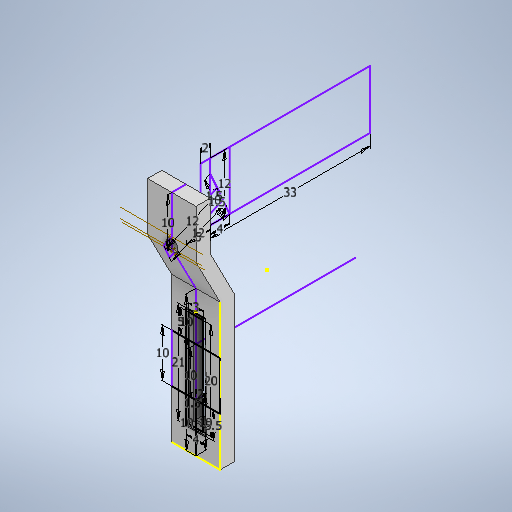
# Autodesk Inventor part: micro_wheel_mount
Saved by Autodesk Inventor 2025 (Build 290162000, 162)
## iProperties
Created: 2025-12-07
Part Number: micro_wheel_mount
Material: Типовые
Document SubType Name: Modeling
Designer: Admin
Density: 1 g/cm^3
Appearance: По умолчанию
Author: Admin
Autodesk Inventor part; units mm, degrees
ref_plane "YZ Plane" through (0, 0, 0) normal (1, 0, 0) x (0, 1, 0)
ref_plane "XZ Plane" through (0, 0, 0) normal (0, 1, 0) x (-1, 0, 0)
ref_plane "XY Plane" through (0, 0, 0) normal (0, 0, 1) x (1, 0, 0)
sketch "Эскиз1" plane through (0, 0, 0) normal (1, 0, 0) x (0, 1, 0)
  line L0 (13.9581, 11.7453) -> (25.9581, 11.7453)
  line L1 (25.9581, 11.7453) -> (25.9581, 13.7453)
  line L2 (25.9581, 13.7453) -> (13.9581, 13.7453)
  line L3 (13.9581, 13.7453) -> (13.9581, 11.7453)
  line L4 (13.9581, 11.7453) -> (13.9581, -21.2547)
  line L5 (13.9581, -21.2547) -> (25.9581, -21.2547)
  line L6 (25.9581, -21.2547) -> (25.9581, 11.7453)
  line L7 (13.9581, 11.7453) -> (13.9581, 7.7453)
  line L8 (13.9581, 7.7453) -> (25.9581, 7.7453)
  line L9 (-6.8518, -18.2547) -> (-6.8518, 11.7453)
  line L10 (-6.8518, 11.7453) -> (-15.825, 11.7453)
  line L11 (-15.825, 11.7453) -> (-15.825, 14.7104)
  line L12 (-15.825, 14.7104) -> (-5.825, 14.7104)
  line L13 (-5.825, 14.7104) -> (-5.825, 11.7453)
  line L14 (-15.825, 14.7104) -> (-25.825, 14.7104)
  line L15 (-25.825, 14.7104) -> (-25.825, 11.7453)
  line L16 (-15.825, 11.7453) -> (-25.825, 11.7453)
  line L17 (-5.825, 14.7104) -> (4.175, 14.7104)
  line L18 (4.175, 14.7104) -> (4.175, 11.7453)
  line L19 (13.9581, 7.7453) -> (23.1232, 11.7453)
  line L20 (23.1232, 11.7453) -> (18.5407, 9.7453)
  line L21 (18.5407, 9.7453) -> (19.9154, 10.3453)
  line L22 (18.5407, 9.7453) -> (17.1659, 9.1453)
  line L23 (19.9154, 10.3453) -> (15.1154, 21.3434)
  line L24 (17.1659, 9.1453) -> (12.3659, 20.1434)
  line L25 (12.3659, 20.1434) -> (15.1154, 21.3434)
  line L26 (13.9581, 11.7453) -> (13.8495, 16.7441)
  line L27 (13.8495, 16.7441) -> (4.175, 11.7453)
  line L28 (4.175, 14.7104) -> (13.7858, 19.6763)
  line L29 (13.7858, 19.6763) -> (23.7858, 19.6763)
  line L30 (23.7858, 19.6763) -> (23.7858, 16.7441)
  line L31 (23.7858, 16.7441) -> (13.8495, 16.7441)
  line L32 (4.175, 11.7453) -> (-5.825, 11.7453)
  line L33 (-5.825, 11.7453) -> (-6.8518, 11.7453)
  point P0 (0, 0)
  dimension "d0" = 12
  dimension "d1" = 2
  dimension "d2" = 33
  dimension "d3" = 4
  dimension "d4" = 10
  dimension "d5" = 10
  dimension "d6" = 10
  dimension "d7" = 10
  dimension "d8" = 1.5
  dimension "d9" = 1.5
  dimension "d10" = 12
  dimension "d11" = 12
  dimension "d12" = 5
  dimension "d13" = 10
  constraints: 68 end point, 11 perpendicular, 11 point on line, 3 horizontal, 2 vertical, 1 midpoint, 1 parallel
  measures "d0" distance of L7.start L6.end
  measures "d1" distance of L6.end L1.end
  measures "d2" distance of L7.start L4.end
  measures "d3" distance of L7.start L7.end
  measures "d4" distance of L11.end L13.start
  measures "d5" distance of L11.end L14.end
  measures "d6" distance of L13.start L18.start
  measures "d7" distance of L7.end L19.end
  measures "d8" distance of L22.start L21.end
  measures "d9" distance of L22.start L22.end
  measures "d10" distance of L21.end L23.end
  measures "d11" distance of L22.end L24.end
  measures "d12" distance of L7.start L31.end
  measures "d13" distance of L29.start L29.end
extrude "Выдавливание1" add sketch "Эскиз1" along normal blind 5 and the other way blind 5 contours L31 L24 L28 L29 L23 | L23 L29 L30 L31 | L27 L18 L28 L24 | L32 L13 L17 L18 | L33 L10 L11 L12 L13 | L11 L16 L15 L14
sketch "Эскиз2" plane through (-5, 4.175, 14.7104) normal (0, -0.459, 0.8884) x (1, 0, 0)
  line L0 (5, 9.6975) -> (5, 12.6658)
  line L1 (5, 12.6658) -> (5, 11.1658)
  circle A0 centre (5, 11.1658) radius 1.25
  point P0 (5, -10.4618)
  dimension "d18" = 1.5
  dimension "d19" = 2.5
  constraints: 4 end point, 1 centre point, 1 coincident, 1 point on line, 1 vertical
  measures "d18" distance of L0.end L1.end
  measures "d19" diameter of A0
sketch "Эскиз3" plane through (-5, -25.825, 14.7104) normal (0, 0, 1) x (1, 0, 0)
  line L0 (0, 0) -> (10, 0) projected
  line L1 (5, 0) -> (5, 10)
  line L2 (5, 10) -> (0, 10)
  line L3 (0, 10) -> (0, 20)
  line L4 (0, 20) -> (10, 20)
  line L5 (10, 20) -> (10, 10)
  line L6 (10, 30) -> (10, 0) projected
  line L7 (5, 10) -> (10, 10)
  line L8 (5, 10) -> (3.5, 10)
  line L9 (3.5, 10) -> (3.5, 20)
  line L10 (3.5, 20) -> (3.5, 25)
  line L11 (3.5, 25) -> (6.5, 25)
  line L12 (6.5, 25) -> (6.5, 5)
  line L13 (6.5, 5) -> (3.5, 5)
  line L14 (3.5, 5) -> (3.5, 10)
  line L15 (5, 10) -> (7, 10)
  line L16 (7, 10) -> (7, 4.5)
  line L17 (7, 4.5) -> (3, 4.5)
  line L18 (3, 4.5) -> (3, 25.5)
  line L19 (3, 25.5) -> (7, 25.5)
  line L20 (7, 25.5) -> (7, 10)
  line L21 (7, 10) -> (7, 4.5)
  line L22 (7, 4.5) -> (5, 4.5)
  line L23 (5, 4.5) -> (5, 10)
  line L24 (6.5, 10) -> (5, 10)
  line L25 (5, 10) -> (5, 5)
  line L26 (5, 5) -> (6.5, 5)
  line L27 (6.5, 5) -> (6.5, 10)
  point P0 (5, 25.825)
  point P1 (5, 5)
  point P2 (5, 5)
  dimension "d22" = 10
  dimension "d23" = 10
  dimension "d24" = 1.5
  dimension "d25" = 5
  dimension "d26" = 3
  dimension "d27" = 20
  dimension "d28" = 2
  dimension "d29" = 5.5
  dimension "d30" = 4
  dimension "d31" = 21
  constraints: 52 end point, 14 perpendicular, 10 point on line, 3 midpoint, 3 parallel, 2 collinear, 1 horizontal, 1 vertical
  measures "d22" distance of L1.start L1.end
  measures "d23" distance of L2.end L3.end
  measures "d24" distance of L1.end L8.end
  measures "d25" distance of L9.end L10.end
  measures "d26" distance of L10.end L11.end
  measures "d27" distance of L11.end L12.end
  measures "d28" distance of L1.end L15.end
  measures "d29" distance of L15.end L16.end
  measures "d30" distance of L16.end L17.end
  measures "d31" distance of L17.end L18.end
extrude "Выдавливание3" cut sketch "Эскиз3" against normal blind 5 contours L13 L14 L2 L1 | L2 L9 L4 L12 L7 | L4 L10 L11 L12
extrude "Выдавливание4" cut sketch "Эскиз3" against normal blind 1.5 contours L17 L18 L2 L14 L13 L1 | L1 L13 L12 L7 L16 L17 | L1 L7 L12 L13 | L7 L12 L4 L20 | L18 L4 L9 L2 | L4 L12 L11 L10 L18 L19 L20
extrude "Выдавливание5" cut sketch "Эскиз3" against normal blind 3 contours L1 L7 L12 L13
extrude "Выдавливание6" cut sketch "Эскиз2" against normal blind 10
